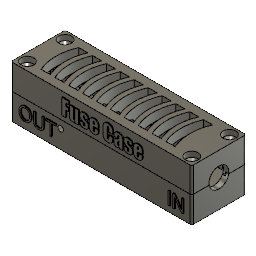
ANL_Fuse_Case (Autodesk Fusion 360 design; units mm, degrees)
Autodesk Fusion 360 part; units mm, degrees
note: some values were not read from the file. Set by a fixed rule: which face or edge a step refers to.
sketch "Skizze1" plane through (0, 0, 0) normal (0, 1, 0) x (1, 0, 0)
  line L0 (50, 15) -> (-50, 15)
  line L1 (-50, 15) -> (-50, -15)
  line L2 (-50, -15) -> (50, -15)
  line L3 (50, -15) -> (50, 15)
  line L4 (50, 15) -> (-50, -15) construction
  line L5 (-50, 15) -> (50, -15) construction
  circle A0 centre (-31, 0) radius 3.1
  line L6 (1.75, 0) -> (22.5, 0)
  line L7 (0, -1.75) -> (0, -22.5)
  circle A1 centre (31, 0) radius 3.1
  dimension "d3" = 30
  dimension "d4" = 100
  dimension "d5" = 6.2
  dimension "d9" = 6.2
  dimension "d10" = 62
  measures "d5" diameter of A0
  measures "d9" diameter of A1
extrude "Extrusion1" add sketch "Skizze1" along normal blind 5 makes body 1
sketch "Skizze3" plane through (0, 5, 0) normal (0, 1, 0) x (-1, 0, 0)
  line L0 (-50, 15) -> (-50, -15)
  line L1 (-50, -15) -> (50, -15)
  line L2 (50, -15) -> (50, 15)
  line L3 (50, 15) -> (-50, 15)
  line L4 (47, -12) -> (-47, -12)
  line L5 (-47, -12) -> (-47, 12)
  line L6 (-47, 12) -> (47, 12)
  line L7 (47, 12) -> (47, -12)
  line L8 (47, -12) -> (-47, 12) construction
  line L9 (-47, -12) -> (47, 12) construction
  circle A0 centre (31, 0) radius 3.1
  circle A1 centre (-31, 0) radius 3.1
  dimension "d17" = 94
  dimension "d18" = 24
extrude "Extrusion3" add sketch "Skizze3" along normal blind 5 contours L0 L1 L2 L3 bodies 1
sketch "Skizze5" plane through (0, 5, 0) normal (0, 1, 0) x (-1, 0, 0)
  line L0 (-47, -12) -> (47, -12)
  line L1 (47, -12) -> (47, 12)
  line L2 (47, 12) -> (-47, 12)
  line L3 (-47, 12) -> (-47, -12)
  circle A0 centre (31, 0) radius 3.1
  circle A1 centre (-31, 0) radius 3.1
  circle A2 centre (31, 0) radius 9
  circle A3 centre (-31, 0) radius 9
  dimension "d25" = 18
  dimension "d26" = 18
  measures "d25" diameter of A2
  measures "d26" diameter of A3
extrude "Extrusion5" add sketch "Skizze5" along normal blind 2 contours A2 | A3 bodies 1
sketch "Skizze6" plane through (0, 0, 0) normal (0, -1, 0) x (1, 0, 0)
  circle A0 centre (-31, 0) radius 3.1
  circle A1 centre (31, 0) radius 3.1
  line L0 (50, -15) -> (50, 15)
  line L1 (50, 15) -> (-50, 15)
  line L2 (-50, 15) -> (-50, -15)
  line L3 (-50, -15) -> (50, -15)
  line L4 (-50, -15) -> (-50, 15)
  line L5 (-50, 15) -> (50, 15)
  line L6 (50, -15) -> (-50, -15)
  line L7 (50, 15) -> (50, -15)
  circle A2 centre (31, 0) radius 3.1
  circle A3 centre (-31, 0) radius 3.1
extrude "Extrusion6" add sketch "Skizze6" along normal blind 3 bodies 1
sketch "Skizze7" plane through (0, -3, 0) normal (0, -1, 0) x (1, 0, 0)
  circle A0 centre (-31, 0) radius 3.1
  circle A1 centre (31, 0) radius 3.1
  line L0 (50, 15) -> (-50, 15)
  line L1 (-50, 15) -> (-50, -15)
  line L2 (-50, -15) -> (50, -15)
  line L3 (50, -15) -> (50, 15)
  line L4 (-33.3094, 4) -> (-35.6188, 0)
  line L5 (-35.6188, 0) -> (-33.3094, -4)
  line L6 (-33.3094, -4) -> (-28.6906, -4)
  line L7 (-28.6906, -4) -> (-26.3812, 0)
  line L8 (-26.3812, 0) -> (-28.6906, 4)
  line L9 (-28.6906, 4) -> (-33.3094, 4)
  line L10 (28.6906, 4) -> (26.3812, 0)
  line L11 (26.3812, 0) -> (28.6906, -4)
  line L12 (28.6906, -4) -> (33.3094, -4)
  line L13 (33.3094, -4) -> (35.6188, 0)
  line L14 (35.6188, 0) -> (33.3094, 4)
  line L15 (33.3094, 4) -> (28.6906, 4)
  dimension "d82" = 8
  dimension "d83" = 8
  measures "d82" distance of L6 L9
  measures "d83" distance of L12 L15
extrude "Extrusion7" cut sketch "Skizze7" against normal blind 5 contours L4 L5 L6 L7 L8 L9 | L10 L11 L12 L13 L14 L15 bodies 1
sketch "Skizze9" plane through (0, 5, 0) normal (0, 1, 0) x (-1, 0, 0)
  circle A0 centre (-31, 0) radius 9
  circle A1 centre (31, 0) radius 9
  line L0 (-47, -12) -> (47, -12)
  line L1 (47, -12) -> (47, 12)
  line L2 (47, 12) -> (-47, 12)
  line L3 (-47, 12) -> (-47, -12)
  line L4 (22, -12) -> (-22, -12)
  line L5 (-22, -12) -> (-22, 12)
  line L6 (-22, 12) -> (22, 12)
  line L7 (22, 12) -> (22, -12)
  line L8 (22, -12) -> (-22, 12) construction
  line L9 (-22, -12) -> (22, 12) construction
  dimension "d35" = 44
extrude "Extrusion9" cut sketch "Skizze9" against normal blind 2 contours L0 L2 L4 L5 L6 L7 bodies 1
sketch "Skizze10" plane through (0, 10, 0) normal (0, 1, 0) x (-1, 0, 0)
  line L0 (-47, 12) -> (47, 12)
  line L1 (47, 12) -> (47, -12)
  line L2 (47, -12) -> (-47, -12)
  line L3 (-47, -12) -> (-47, 12)
  line L4 (50, 15) -> (-50, 15)
  line L5 (-50, 15) -> (-50, -15)
  line L6 (-50, -15) -> (50, -15)
  line L7 (50, -15) -> (50, 15)
  line L8 (48.6, -13.6) -> (-48.6, -13.6)
  line L9 (-48.6, -13.6) -> (-48.6, 13.6)
  line L10 (-48.6, 13.6) -> (48.6, 13.6)
  line L11 (48.6, 13.6) -> (48.6, -13.6)
  line L12 (48.6, -13.6) -> (-48.6, 13.6) construction
  line L13 (-48.6, -13.6) -> (48.6, 13.6) construction
  dimension "d92" = 27.2
  dimension "d93" = 97.2
  measures "d92" distance of L8 L10
  measures "d93" distance of L9 L11
extrude "Extrusion10" add sketch "Skizze10" along normal blind 1.5 contours L4 L5 L6 L7 bodies 1
sketch "Skizze11" plane through (0, 11.5, 0) normal (0, 1, 0) x (-1, 0, 0)
  line L0 (-48.6, 13.6) -> (48.6, 13.6)
  line L1 (48.6, 13.6) -> (48.6, -13.6)
  line L2 (48.6, -13.6) -> (-48.6, -13.6)
  line L3 (-48.6, -13.6) -> (-48.6, 13.6)
  line L4 (50, -15) -> (50, 15)
  line L5 (50, 15) -> (-50, 15)
  line L6 (-50, 15) -> (-50, -15)
  line L7 (-50, -15) -> (50, -15)
  line L8 (50, -15) -> (-50, -15)
  line L9 (-50, -15) -> (-50, 15)
  line L10 (-50, 15) -> (50, 15)
  line L11 (50, 15) -> (50, -15)
  line L12 (50, -15) -> (-50, 15) construction
  line L13 (-50, -15) -> (50, 15) construction
  line L14 (47, -12) -> (-47, -12)
  line L15 (-47, -12) -> (-47, 12)
  line L16 (-47, 12) -> (47, 12)
  line L17 (47, 12) -> (47, -12)
  line L18 (47, -12) -> (-47, 12) construction
  line L19 (-47, -12) -> (47, 12) construction
extrude "Extrusion11" add sketch "Skizze11" along normal blind 9 separate body contours L0 L1 L2 L3 | L4 L5 L6 L7 L8 L9 L10 L11 makes body 2
sketch "Skizze12" plane through (0, 11.5, 0) normal (0, -1, 0) x (1, 0, 0)
  line L0 (-47, 12) -> (47, 12)
  line L1 (47, 12) -> (47, -12)
  line L2 (47, -12) -> (-47, -12)
  line L3 (-47, -12) -> (-47, 12)
  line L4 (50, 15) -> (-50, 15)
  line L5 (-50, 15) -> (-50, -15)
  line L6 (-50, -15) -> (50, -15)
  line L7 (50, -15) -> (50, 15)
  line L8 (-48.25, 13.25) -> (48.25, 13.25)
  line L9 (48.25, 13.25) -> (48.25, -13.25)
  line L10 (48.25, -13.25) -> (-48.25, -13.25)
  line L11 (-48.25, -13.25) -> (-48.25, 13.25)
  line L12 (-48.25, 13.25) -> (48.25, -13.25) construction
  line L13 (48.25, 13.25) -> (-48.25, -13.25) construction
  dimension "d42" = 96.5
  dimension "d94" = 26.5
extrude "Extrusion12" add sketch "Skizze12" along normal blind 1 contours L8 L9 L10 L11 bodies 2
sketch "Skizze13" plane through (-50, 0, 0) normal (-1, 0, 0) x (0, 0, 1)
  line L0 (15, -3) -> (15, 11.5)
  line L1 (15, 11.5) -> (-15, 11.5)
  line L2 (-15, 11.5) -> (-15, -3)
  line L3 (-15, -3) -> (15, -3)
  line L4 (-12, 5) -> (12, 5)
  line L5 (0, 1.75) -> (0, 22.5)
  circle A0 centre (0, 12.5) radius 5.5
  dimension "d45" = 11
  dimension "d46" = 7.5
  measures "d45" diameter of A0
  measures "d46" distance of L4
extrude "Extrusion13" cut sketch "Skizze13" against normal blind 100 contours L1 L5 A0 | L1 L5 A0 | L1 L5 A0 | L1 L5 A0 bodies 1 2
sketch "Skizze14" plane through (0, 5, 0) normal (0, 1, 0) x (-1, 0, 0)
  line L0 (22, -12) -> (47, -12)
  line L1 (47, -12) -> (47, 12)
  line L2 (47, 12) -> (22, 12)
  circle A0 centre (31, 0) radius 9
  arc A1 (47, -7) -> (42, -12) centre (47, -12) ccw
  arc A2 (42, 12) -> (47, 7) centre (47, 12) ccw
  arc A3 (-42, -12) -> (-47, -7) centre (-47, -12) ccw
  line L3 (-47, -12) -> (47, -12)
  line L4 (-47, -5.1235) -> (-47, -12)
  arc A4 (-47, 7) -> (-42, 12) centre (-47, 12) ccw
  line L5 (-47, -12) -> (-47, 12)
  line L6 (-22, 12) -> (-47, 12)
  line L7 (22, 0) -> (22, -12)
  line L8 (22, 12) -> (22, 0)
  dimension "d49" = 5
  dimension "d50" = 5
  dimension "d51" = 5
  dimension "d52" = 5
  measures "d49" radius of A1
  measures "d50" radius of A2
  measures "d51" radius of A3
  measures "d52" radius of A4
extrude "Extrusion14" add sketch "Skizze14" along normal blind 5 contours L0 L1 A1 L3 | L1 L2 A2 | A3 L3 L4 L5 | A4 L5 L6 bodies 1
sketch "Skizze15" plane through (0, 10, 0) normal (0, 1, 0) x (-1, 0, 0)
  line L0 (-47, -4.899) -> (-48.6, -4.899)
  line L1 (-48.6, -4.899) -> (-48.6, -13.6)
  line L2 (-48.6, -13.6) -> (48.6, -13.6)
  line L3 (48.6, -13.6) -> (48.6, -4.899)
  line L4 (48.6, -4.899) -> (47, -4.899)
  line L5 (47, -4.899) -> (47, -7)
  arc A0 (47, -7) -> (42, -12) centre (47, -12) ccw
  line L6 (42, -12) -> (-42, -12)
  arc A1 (-42, -12) -> (-47, -7) centre (-47, -12) ccw
  line L7 (-47, -7) -> (-47, -4.899)
  circle A2 centre (45.4, -10.4) radius 1.6
  line L8 (47, -12) -> (-47, -12)
  line L9 (47, 12) -> (47, -12)
  circle A3 centre (45.4, 10.4) radius 1.6
  line L10 (-47, 12) -> (47, 12)
  circle A4 centre (-45.4, -10.4) radius 1.6
  line L11 (-47, -12) -> (-47, 12)
  circle A5 centre (-45.4, 10.4) radius 1.6
  dimension "d55" = 3.2
  dimension "d56" = 3.2
  dimension "d57" = 3.2
  dimension "d58" = 3.2
  measures "d55" diameter of A2
  measures "d56" diameter of A3
  measures "d57" diameter of A4
  measures "d58" diameter of A5
extrude "Extrusion15" cut sketch "Skizze15" against normal blind 13 contours A5 | A4 | A3 | A2 bodies 1
sketch "Skizze16" plane through (0, -3, 0) normal (0, -1, 0) x (1, 0, 0)
  circle A0 centre (-45.4, 10.4) radius 1.6
  circle A1 centre (45.4, -10.4) radius 1.6
  circle A2 centre (-45.4, -10.4) radius 1.6
  circle A3 centre (45.4, 10.4) radius 1.6
  line L0 (26.3812, 0) -> (28.6906, 4)
  line L1 (28.6906, 4) -> (33.3094, 4)
  line L2 (33.3094, 4) -> (35.6188, 0)
  line L3 (35.6188, 0) -> (33.3094, -4)
  line L4 (33.3094, -4) -> (28.6906, -4)
  line L5 (28.6906, -4) -> (26.3812, 0)
  line L6 (-35.6188, 0) -> (-33.3094, 4)
  line L7 (-33.3094, 4) -> (-28.6906, 4)
  line L8 (-28.6906, 4) -> (-26.3812, 0)
  line L9 (-26.3812, 0) -> (-28.6906, -4)
  line L10 (-28.6906, -4) -> (-33.3094, -4)
  line L11 (-33.3094, -4) -> (-35.6188, 0)
  line L12 (50, 15) -> (-50, 15)
  line L13 (-50, 15) -> (-50, -15)
  line L14 (-50, -15) -> (50, -15)
  line L15 (50, -15) -> (50, 15)
  line L16 (-47.0166, 13.2) -> (-48.6332, 10.4)
  line L17 (-48.6332, 10.4) -> (-47.0166, 7.6)
  line L18 (-47.0166, 7.6) -> (-43.7834, 7.6)
  line L19 (-43.7834, 7.6) -> (-42.1668, 10.4)
  line L20 (-42.1668, 10.4) -> (-43.7834, 13.2)
  line L21 (-43.7834, 13.2) -> (-47.0166, 13.2)
  line L22 (-47.0166, -7.6) -> (-48.6332, -10.4)
  line L23 (-48.6332, -10.4) -> (-47.0166, -13.2)
  line L24 (-47.0166, -13.2) -> (-43.7834, -13.2)
  line L25 (-43.7834, -13.2) -> (-42.1668, -10.4)
  line L26 (-42.1668, -10.4) -> (-43.7834, -7.6)
  line L27 (-43.7834, -7.6) -> (-47.0166, -7.6)
  line L28 (43.7834, -7.6) -> (42.1668, -10.4)
  line L29 (42.1668, -10.4) -> (43.7834, -13.2)
  line L30 (43.7834, -13.2) -> (47.0166, -13.2)
  line L31 (47.0166, -13.2) -> (48.6332, -10.4)
  line L32 (48.6332, -10.4) -> (47.0166, -7.6)
  line L33 (47.0166, -7.6) -> (43.7834, -7.6)
  line L34 (43.7834, 13.2) -> (42.1668, 10.4)
  line L35 (42.1668, 10.4) -> (43.7834, 7.6)
  line L36 (43.7834, 7.6) -> (47.0166, 7.6)
  line L37 (47.0166, 7.6) -> (48.6332, 10.4)
  line L38 (48.6332, 10.4) -> (47.0166, 13.2)
  line L39 (47.0166, 13.2) -> (43.7834, 13.2)
  dimension "d88" = 5.6
  dimension "d89" = 5.6
  dimension "d90" = 5.6
  dimension "d91" = 5.6
  measures "d88" distance of L18 L21
  measures "d89" distance of L24 L27
  measures "d90" distance of L36 L39
  measures "d91" distance of L30 L33
extrude "Extrusion16" cut sketch "Skizze16" against normal blind 3 contours L16 L17 L18 L19 L20 L21 | L22 L23 L24 L25 L26 L27 | L28 L29 L30 L31 L32 L33 | L34 L35 L36 L37 L38 L39 bodies 1
sketch "Skizze17" plane through (0, 20.5, 0) normal (0, 1, 0) x (-1, 0, 0)
  line L0 (-47, 12) -> (47, 12)
  line L1 (47, 12) -> (47, -12)
  line L2 (47, -12) -> (-47, -12)
  line L3 (-47, -12) -> (-47, 12)
  line L4 (50, 15) -> (-50, 15)
  line L5 (-50, 15) -> (-50, -15)
  line L6 (-50, -15) -> (50, -15)
  line L7 (50, -15) -> (50, 15)
extrude "Extrusion17" add sketch "Skizze17" along normal blind 5 contours L0 L1 L2 L3 | L4 L5 L6 L7 bodies 2
sketch "Skizze18" plane through (0, 25.5, 0) normal (0, 1, 0) x (-1, 0, 0)
  line L0 (50, -15) -> (50, 15)
  line L1 (50, 15) -> (-50, 15)
  line L2 (-50, 15) -> (-50, -15)
  line L3 (-50, -15) -> (50, -15)
  circle A0 centre (45.4, 10.4) radius 1.6
  circle A1 centre (45.4, -10.4) radius 1.6
  circle A2 centre (-45.4, 10.4) radius 1.6
  circle A3 centre (-45.4, 10.4) radius 1.6
  circle A4 centre (-45.4, -10.4) radius 1.6
  circle A5 centre (45.4, -10.4) radius 3.5
  circle A6 centre (45.4, 10.4) radius 3.5
  circle A7 centre (-45.4, 10.4) radius 3.5
  circle A8 centre (-45.4, -10.4) radius 3.5
  dimension "d65" = 7
  dimension "d66" = 7
  dimension "d67" = 7
  dimension "d68" = 7
  measures "d65" diameter of A5
  measures "d66" diameter of A6
  measures "d67" diameter of A7
  measures "d68" diameter of A8
extrude "Extrusion18" cut sketch "Skizze18" against normal blind 3 contours A5 | A6 | A7 | A8 bodies 2
extrude "Extrusion19" cut 4 faces at (-45.7325, 25.5, -11.1314) (-45.791, 25.5, 11.0772) (45.009, 25.5, -9.7228) (45.009, 25.5, 11.0772) along direction (0, -1, 0) blind 5 on bodies 2 bodies 2
sketch "Skizze19" plane through (0, 20.5, 0) normal (0, -1, 0) x (1, 0, 0)
  arc A0 (47, -10.4) -> (45.4, -12) centre (45.4, -10.4) ccw
  line L0 (47, -10.4) -> (47, 10.4)
  arc A1 (45.4, 12) -> (47, 10.4) centre (45.4, 10.4) ccw
  line L1 (45.4, 12) -> (-45.4, 12)
  arc A2 (-47, 10.4) -> (-45.4, 12) centre (-45.4, 10.4) ccw
  line L2 (-47, 10.4) -> (-47, -10.4)
  arc A3 (-45.4, -12) -> (-47, -10.4) centre (-45.4, -10.4) ccw
  line L3 (-45.4, -12) -> (45.4, -12)
  arc A4 (-42, -12) -> (-47, -7) centre (-47, -12) ccw
  arc A5 (-47, 7) -> (-42, 12) centre (-47, 12) ccw
  arc A6 (47, -7) -> (42, -12) centre (47, -12) ccw
  arc A7 (42, 12) -> (47, 7) centre (47, 12) ccw
extrude "Extrusion20" add sketch "Skizze19" 4 faces at (46.6857, 20.5, -11.6857) (46.6857, 20.5, 11.6857) (-46.6857, 20.5, -11.6857) (-46.6857, 20.5, 11.6857) along normal blind 10 contours A0 L0 L3 A6 | L0 A1 L1 A7 | L2 A3 L3 A4 | L1 A2 L2 A5 on bodies 2 bodies 2
sketch "Skizze20" plane through (0, 25.5, 0) normal (0, 1, 0) x (-1, 0, 0)
  circle A0 centre (45.4, 10.4) radius 3.5
  circle A1 centre (-45.4, -10.4) radius 3.5
  circle A2 centre (45.4, -10.4) radius 3.5
  circle A3 centre (-45.4, 10.4) radius 3.5
  line L0 (50, -15) -> (50, 15)
  line L1 (50, 15) -> (-50, 15)
  line L2 (-50, 15) -> (-50, -15)
  line L3 (-50, -15) -> (50, -15)
  arc A4 (32.8458, -10.3624) -> (32.8316, 10.3949) centre (9, 0) ccw
  arc A5 (37.8458, -10.3624) -> (37.815, 10.433) centre (14, 0) ccw
  circle A6 centre (31, 0) radius 9
  line L4 (37.8458, -10.3624) -> (32.8458, -10.3624)
  line L5 (37.815, 10.433) -> (32.8316, 10.3949)
  arc A7 (30.1791, -10.3624) -> (30.1483, 10.433) centre (6.3333, 0) ccw
  arc A8 (25.1791, -10.3624) -> (25.165, 10.3949) centre (1.3333, 0) ccw
  line L6 (30.1791, -10.3624) -> (25.1791, -10.3624)
  line L7 (30.1483, 10.433) -> (25.165, 10.3949)
  arc A9 (22.5124, -10.3624) -> (22.4816, 10.433) centre (-1.3333, 0) ccw
  arc A10 (17.5124, -10.3624) -> (17.4983, 10.3949) centre (-6.3333, 0) ccw
  line L8 (22.5124, -10.3624) -> (17.5124, -10.3624)
  line L9 (22.4816, 10.433) -> (17.4983, 10.3949)
  arc A11 (14.8458, -10.3624) -> (14.815, 10.433) centre (-9, 0) ccw
  arc A12 (9.8458, -10.3624) -> (9.8316, 10.3949) centre (-14, 0) ccw
  line L10 (14.8458, -10.3624) -> (9.8458, -10.3624)
  line L11 (14.815, 10.433) -> (9.8316, 10.3949)
  arc A13 (7.1791, -10.3624) -> (7.1483, 10.433) centre (-16.6667, 0) ccw
  arc A14 (2.1791, -10.3624) -> (2.165, 10.3949) centre (-21.6667, 0) ccw
  line L12 (7.1791, -10.3624) -> (2.1791, -10.3624)
  line L13 (7.1483, 10.433) -> (2.165, 10.3949)
  arc A15 (-0.4876, -10.3624) -> (-0.5184, 10.433) centre (-24.3333, 0) ccw
  arc A16 (-5.4876, -10.3624) -> (-5.5017, 10.3949) centre (-29.3333, 0) ccw
  line L14 (-0.4876, -10.3624) -> (-5.4876, -10.3624)
  line L15 (-0.5184, 10.433) -> (-5.5017, 10.3949)
  arc A17 (-8.1542, -10.3624) -> (-8.185, 10.433) centre (-32, 0) ccw
  arc A18 (-13.1542, -10.3624) -> (-13.1684, 10.3949) centre (-37, 0) ccw
  line L16 (-8.1542, -10.3624) -> (-13.1542, -10.3624)
  line L17 (-8.185, 10.433) -> (-13.1684, 10.3949)
  arc A19 (-15.8209, -10.3624) -> (-15.8517, 10.433) centre (-39.6667, 0) ccw
  arc A20 (-20.8209, -10.3624) -> (-20.835, 10.3949) centre (-44.6667, 0) ccw
  line L18 (-15.8209, -10.3624) -> (-20.8209, -10.3624)
  line L19 (-15.8517, 10.433) -> (-20.835, 10.3949)
  arc A21 (-23.4876, -10.3624) -> (-23.5184, 10.433) centre (-47.3333, 0) ccw
  arc A22 (-28.4876, -10.3624) -> (-28.5017, 10.3949) centre (-52.3333, 0) ccw
  line L20 (-23.4876, -10.3624) -> (-28.4876, -10.3624)
  line L21 (-23.5184, 10.433) -> (-28.5017, 10.3949)
  arc A23 (-31.1542, -10.3624) -> (-31.185, 10.433) centre (-55, 0) ccw
  arc A24 (-36.1542, -10.3624) -> (-36.1684, 10.3949) centre (-60, 0) ccw
  line L22 (-31.1542, -10.3624) -> (-36.1542, -10.3624)
  line L23 (-31.185, 10.433) -> (-36.1684, 10.3949)
  dimension "d77" = -69
  dimension "d78" = 0
extrude "Extrusion21" cut sketch "Skizze20" against normal blind 5 contours A4 A5 A6 L4 | A4 A6 | A4 A5 A6 L5 | A6 A7 A8 L6 | A6 A7 A8 | A6 A7 A8 L7 | A6 A9 A10 L8 L9 | A6 A9 | A11 A12 L10 L11 | A13 A14 L12 L13 | A15 A16 L14 L15 | A17 A18 L16 L17 | A19 A20 L18 L19 | A21 A22 L20 L21 | A23 A24 L22 L23 bodies 2
fillet "Abrundung1" radius 1 8 edges at (-50, 4.25, 15) (50, 4.25, 15) (50, 4.25, -15) (-50, 4.25, -15) (-50, 18.5, 15) (50, 18.5, 15) (50, 18.5, -15) (-50, 18.5, -15) on bodies 1 2
sketch "Skizze21" plane through (0, 2, 0) normal (0, -1, 0) x (1, 0, 0)
  circle A0 centre (-31, 0) radius 3.1
  line L0 (-28.6906, 4) -> (-33.3094, 4)
  line L1 (-33.3094, 4) -> (-35.6188, 0)
  line L2 (-35.6188, 0) -> (-33.3094, -4)
  line L3 (-33.3094, -4) -> (-28.6906, -4)
  line L4 (-28.6906, -4) -> (-26.3812, 0)
  line L5 (-26.3812, 0) -> (-28.6906, 4)
  circle A1 centre (-31, 0) radius 2.6
  circle A2 centre (31, 0) radius 2.6
  circle A3 centre (31, 0) radius 3.1
  dimension "d84" = 5.2
  dimension "d85" = 5.2
  measures "d84" diameter of A1
  measures "d85" diameter of A2
extrude "Extrusion22" add sketch "Skizze21" against normal blind 5 contours A0 | A3 bodies 1
sketch "Skizze22" plane through (0, 3, 0) normal (0, 1, 0) x (-1, 0, 0)
  line L0 (22, 12) -> (-22, 12)
  line L1 (-22, 12) -> (-22, -12)
  line L2 (-22, -12) -> (22, -12)
  line L3 (22, -12) -> (22, 12)
  line L4 (22, -12) -> (-22, -12)
  line L5 (-22, -12) -> (-22, -11)
  line L6 (-22, -11) -> (22, -11)
  line L7 (22, -11) -> (22, -12)
  line L8 (22, 12) -> (-22, 12)
  line L9 (-22, 12) -> (-22, 11)
  line L10 (-22, 11) -> (22, 11)
  line L11 (22, 11) -> (22, 12)
  dimension "d95" = 24
  dimension "d96" = 1
  dimension "d97" = 1
  measures "d95" distance of L0 L4
  measures "d96" distance of L4 L6
  measures "d97" distance of L8 L10
extrude "Extrusion23" add sketch "Skizze22" along normal blind 2 contours L0 L1 L3 L8 L9 L10 L11 | L1 L2 L3 L4 L5 L6 L7 bodies 1
sketch "Skizze24" plane through (0, 0, 15) normal (0, 0, 1) x (1, 0, 0)
  line L0 (49, 11.5) -> (49, 25.5)
  line L1 (49, 25.5) -> (-49, 25.5)
  line L2 (-49, 25.5) -> (-49, 11.5)
  line L3 (-49, 11.5) -> (49, 11.5)
  line L4 (-21.3454, 14.0591) -> (23.181, 14.0591) construction
  line L5 (23.181, 14.0591) -> (23.181, 25.0591) construction
  line L6 (23.181, 25.0591) -> (-21.3454, 25.0591) construction
  line L7 (-21.3454, 25.0591) -> (-21.3454, 14.0591) construction
  text T0 "Fuse Case" font "Impact" height 11 align ink ink in box 0 x 0 at (-21.3454, 14.0591) x (1, 0) y (0, 1) spacing 1 height is em
extrude "Extrusion24" add sketch "Skizze24" along normal blind 0.5 text T0 bodies 2
sketch "Skizze25" plane through (0, 7, 0) normal (0, 1, 0) x (-1, 0, 0)
  circle A0 centre (31, 0) radius 2.6
  circle A1 centre (31, 0) radius 9
  line L0 (33.3094, -4) -> (35.6188, 0)
  line L1 (35.6188, 0) -> (33.3094, 4)
  line L2 (33.3094, 4) -> (28.6906, 4)
  line L3 (28.6906, 4) -> (26.3812, 0)
  line L4 (26.3812, 0) -> (28.6906, -4)
  line L5 (28.6906, -4) -> (33.3094, -4)
  line L6 (-28.6906, -4) -> (-26.3812, 0)
  line L7 (-26.3812, 0) -> (-28.6906, 4)
  line L8 (-28.6906, 4) -> (-33.3094, 4)
  line L9 (-33.3094, 4) -> (-35.6188, 0)
  line L10 (-35.6188, 0) -> (-33.3094, -4)
  line L11 (-33.3094, -4) -> (-28.6906, -4)
  dimension "d102" = 8
  dimension "d103" = 8
  measures "d102" distance of L2 L5
  measures "d103" distance of L8 L11
extrude "Extrusion25" cut sketch "Skizze25" against normal blind 5 contours L0 L1 L2 L3 L4 L5 | L6 L7 L8 L9 L10 L11 bodies 1
sketch "Skizze26" plane through (0, -3, 0) normal (0, -1, 0) x (1, 0, 0)
  line L0 (-48.6332, -10.4) -> (-47.0166, -7.6)
  line L1 (-47.0166, -7.6) -> (-43.7834, -7.6)
  line L2 (-43.7834, -7.6) -> (-42.1668, -10.4)
  line L3 (-42.1668, -10.4) -> (-43.7834, -13.2)
  line L4 (-43.7834, -13.2) -> (-47.0166, -13.2)
  line L5 (-47.0166, -13.2) -> (-48.6332, -10.4)
  line L6 (42.1668, 10.4) -> (43.7834, 13.2)
  line L7 (43.7834, 13.2) -> (47.0166, 13.2)
  line L8 (47.0166, 13.2) -> (48.6332, 10.4)
  line L9 (48.6332, 10.4) -> (47.0166, 7.6)
  line L10 (47.0166, 7.6) -> (43.7834, 7.6)
  line L11 (43.7834, 7.6) -> (42.1668, 10.4)
  line L12 (-48.6332, 10.4) -> (-47.0166, 13.2)
  line L13 (-47.0166, 13.2) -> (-43.7834, 13.2)
  line L14 (-43.7834, 13.2) -> (-42.1668, 10.4)
  line L15 (-42.1668, 10.4) -> (-43.7834, 7.6)
  line L16 (-43.7834, 7.6) -> (-47.0166, 7.6)
  line L17 (-47.0166, 7.6) -> (-48.6332, 10.4)
  line L18 (42.1668, -10.4) -> (43.7834, -7.6)
  line L19 (43.7834, -7.6) -> (47.0166, -7.6)
  line L20 (47.0166, -7.6) -> (48.6332, -10.4)
  line L21 (48.6332, -10.4) -> (47.0166, -13.2)
  line L22 (47.0166, -13.2) -> (43.7834, -13.2)
  line L23 (43.7834, -13.2) -> (42.1668, -10.4)
  line L24 (26.3812, 0) -> (28.6906, 4)
  line L25 (28.6906, 4) -> (33.3094, 4)
  line L26 (33.3094, 4) -> (35.6188, 0)
  line L27 (35.6188, 0) -> (33.3094, -4)
  line L28 (33.3094, -4) -> (28.6906, -4)
  line L29 (28.6906, -4) -> (26.3812, 0)
  line L30 (-35.6188, 0) -> (-33.3094, 4)
  line L31 (-33.3094, 4) -> (-28.6906, 4)
  line L32 (-28.6906, 4) -> (-26.3812, 0)
  line L33 (-26.3812, 0) -> (-28.6906, -4)
  line L34 (-28.6906, -4) -> (-33.3094, -4)
  line L35 (-33.3094, -4) -> (-35.6188, 0)
  arc A0 (-50, -14) -> (-49, -15) centre (-49, -14) ccw
  line L36 (-49, -15) -> (49, -15)
  arc A1 (49, -15) -> (50, -14) centre (49, -14) ccw
  line L37 (50, -14) -> (50, 14)
  arc A2 (50, 14) -> (49, 15) centre (49, 14) ccw
  line L38 (49, 15) -> (-49, 15)
  arc A3 (-49, 15) -> (-50, 14) centre (-49, 14) ccw
  line L39 (-50, 14) -> (-50, -14)
  circle A4 centre (-31, 0) radius 2.6
  line L40 (-28.6906, 4) -> (-33.3094, 4)
  line L41 (-33.3094, 4) -> (-35.6188, 0)
  line L42 (-35.6188, 0) -> (-33.3094, -4)
  line L43 (-33.3094, -4) -> (-28.6906, -4)
  line L44 (-28.6906, -4) -> (-26.3812, 0)
  line L45 (-26.3812, 0) -> (-28.6906, 4)
  circle A5 centre (31, 0) radius 2.6
  line L46 (33.3094, 4) -> (28.6906, 4)
  line L47 (28.6906, 4) -> (26.3812, 0)
  line L48 (26.3812, 0) -> (28.6906, -4)
  line L49 (28.6906, -4) -> (33.3094, -4)
  line L50 (33.3094, -4) -> (35.6188, 0)
  line L51 (35.6188, 0) -> (33.3094, 4)
extrude "Extrusion26" add sketch "Skizze26" against normal blind 5 contours L24 L25 L26 L27 L28 L29 L46 L47 L48 L49 L50 L51 | L30 L31 L32 L33 L34 L35 L40 L41 L42 L43 L44 L45 bodies 1
extrude "Extrusion27" cut 2 faces at (26.2119, 7, 3.0233) (-36.0123, 7, 2.635) along direction (0, -1, 0) blind 1 on bodies 1 bodies 1
sketch "Skizze28" plane through (0, 0, 15) normal (0, 0, 1) x (1, 0, 0)
  line L0 (49, -3) -> (49, 11.5)
  line L1 (49, 11.5) -> (-49, 11.5)
  line L2 (-49, 11.5) -> (-49, -3)
  line L3 (-49, -3) -> (49, -3)
  line L4 (37.4033, 0.5851) -> (45.6504, 0.5851) construction
  line L5 (45.6504, 0.5851) -> (45.6504, 10.5851) construction
  line L6 (45.6504, 10.5851) -> (37.4033, 10.5851) construction
  line L7 (37.4033, 10.5851) -> (37.4033, 0.5851) construction
  line L8 (-45.0165, 1.0191) -> (-24.5917, 1.0191) construction
  line L9 (-24.5917, 1.0191) -> (-24.5917, 11.0191) construction
  line L10 (-24.5917, 11.0191) -> (-45.0165, 11.0191) construction
  line L11 (-45.0165, 11.0191) -> (-45.0165, 1.0191) construction
  text T0 "IN" font "Arial" height 10 align ink ink in box 0 x 0 at (37.4033, 0.5851) x (1, 0) y (0, 1) spacing 1 height is em
  text T1 "OUT" font "Arial" height 10 align ink ink in box 0 x 0 at (-45.0165, 1.0191) x (1, 0) y (0, 1) spacing 1 height is em
extrude "Extrusion28" add sketch "Skizze28" along normal blind 0.5 text T0 T1 bodies 1
sketch "Skizze29" plane through (0, 0, -12) normal (0, 0, 1) x (1, 0, 0)
  line L0 (-42, 5) -> (42, 5)
  line L1 (42, 5) -> (42, 10)
  line L2 (42, 10) -> (-42, 10)
  line L3 (-42, 10) -> (-42, 5)
  circle A0 centre (-25, 7.5) radius 1.5
  dimension "d112" = 3
  dimension "d113" = 2.5
  measures "d112" diameter of A0
  measures "d113" distance of L0
extrude "Extrusion29" cut sketch "Skizze29" against normal blind 3 contours A0 bodies 1
sketch "Skizze30" plane through (0, 20.5, 0) normal (0, -1, 0) x (1, 0, 0)
  line L0 (31.185, 10.433) -> (36.1684, 10.3949)
  arc A0 (36.1684, 10.3949) -> (36.1542, -10.3624) centre (60, 0) ccw
  line L1 (36.1542, -10.3624) -> (31.1542, -10.3624)
  arc A1 (31.185, 10.433) -> (31.1542, -10.3624) centre (55, 0) ccw
  line L2 (0.5184, 10.433) -> (5.5017, 10.3949)
  arc A2 (5.5017, 10.3949) -> (5.4876, -10.3624) centre (29.3333, 0) ccw
  line L3 (5.4876, -10.3624) -> (0.4876, -10.3624)
  arc A3 (0.5184, 10.433) -> (0.4876, -10.3624) centre (24.3333, 0) ccw
  line L4 (-22.4816, 10.433) -> (-17.4983, 10.3949)
  arc A4 (-17.4983, 10.3949) -> (-17.5124, -10.3624) centre (6.3333, 0) ccw
  line L5 (-17.5124, -10.3624) -> (-22.5124, -10.3624)
  arc A5 (-22.4816, 10.433) -> (-22.5124, -10.3624) centre (1.3333, 0) ccw
  line L6 (8.185, 10.433) -> (13.1684, 10.3949)
  arc A6 (13.1684, 10.3949) -> (13.1542, -10.3624) centre (37, 0) ccw
  line L7 (13.1542, -10.3624) -> (8.1542, -10.3624)
  arc A7 (8.185, 10.433) -> (8.1542, -10.3624) centre (32, 0) ccw
  line L8 (-37.815, 10.433) -> (-32.8316, 10.3949)
  arc A8 (-32.8316, 10.3949) -> (-32.8458, -10.3624) centre (-9, 0) ccw
  line L9 (-32.8458, -10.3624) -> (-37.8458, -10.3624)
  arc A9 (-37.815, 10.433) -> (-37.8458, -10.3624) centre (-14, 0) ccw
  line L10 (23.5184, 10.433) -> (28.5017, 10.3949)
  arc A10 (28.5017, 10.3949) -> (28.4876, -10.3624) centre (52.3333, 0) ccw
  line L11 (28.4876, -10.3624) -> (23.4876, -10.3624)
  arc A11 (23.5184, 10.433) -> (23.4876, -10.3624) centre (47.3333, 0) ccw
  line L12 (-7.1483, 10.433) -> (-2.165, 10.3949)
  arc A12 (-2.165, 10.3949) -> (-2.1791, -10.3624) centre (21.6667, 0) ccw
  line L13 (-2.1791, -10.3624) -> (-7.1791, -10.3624)
  arc A13 (-7.1483, 10.433) -> (-7.1791, -10.3624) centre (16.6667, 0) ccw
  line L14 (-14.815, 10.433) -> (-9.8316, 10.3949)
  arc A14 (-9.8316, 10.3949) -> (-9.8458, -10.3624) centre (14, 0) ccw
  line L15 (-9.8458, -10.3624) -> (-14.8458, -10.3624)
  arc A15 (-14.815, 10.433) -> (-14.8458, -10.3624) centre (9, 0) ccw
  line L16 (15.8517, 10.433) -> (20.835, 10.3949)
  arc A16 (20.835, 10.3949) -> (20.8209, -10.3624) centre (44.6667, 0) ccw
  line L17 (20.8209, -10.3624) -> (15.8209, -10.3624)
  arc A17 (15.8517, 10.433) -> (15.8209, -10.3624) centre (39.6667, 0) ccw
  line L18 (-30.1483, 10.433) -> (-25.165, 10.3949)
  arc A18 (-25.165, 10.3949) -> (-25.1791, -10.3624) centre (-1.3333, 0) ccw
  line L19 (-25.1791, -10.3624) -> (-30.1791, -10.3624)
  arc A19 (-30.1483, 10.433) -> (-30.1791, -10.3624) centre (-6.3333, 0) ccw
  arc A20 (-47, 7) -> (-42, 12) centre (-47, 12) ccw
  line L20 (-47, 7) -> (-47, -7)
  arc A21 (-42, -12) -> (-47, -7) centre (-47, -12) ccw
  line L21 (-42, -12) -> (42, -12)
  arc A22 (47, -7) -> (42, -12) centre (47, -12) ccw
  line L22 (47, -7) -> (47, 7)
  arc A23 (42, 12) -> (47, 7) centre (47, 12) ccw
  line L23 (42, 12) -> (-42, 12)
  arc A24 (-9.8316, 10.3949) -> (-9.8458, -10.3624) centre (14, 0) ccw
  arc A25 (-50, -14) -> (-49, -15) centre (-49, -14) ccw
  line L24 (-50, -14) -> (-50, 14)
  arc A26 (-49, 15) -> (-50, 14) centre (-49, 14) ccw
  line L25 (-49, 15) -> (49, 15)
  arc A27 (50, 14) -> (49, 15) centre (49, 14) ccw
  line L26 (50, 14) -> (50, -14)
  arc A28 (49, -15) -> (50, -14) centre (49, -14) ccw
  line L27 (49, -15) -> (-49, -15)
  line L28 (36.1684, 10.3949) -> (31.185, 10.433)
  arc A29 (31.185, 10.433) -> (31.1542, -10.3624) centre (55, 0) ccw
  line L29 (31.1542, -10.3624) -> (36.1542, -10.3624)
  arc A30 (36.1684, 10.3949) -> (36.1542, -10.3624) centre (60, 0) ccw
  line L30 (5.5017, 10.3949) -> (0.5184, 10.433)
  arc A31 (0.5184, 10.433) -> (0.4876, -10.3624) centre (24.3333, 0) ccw
  line L31 (0.4876, -10.3624) -> (5.4876, -10.3624)
  arc A32 (5.5017, 10.3949) -> (5.4876, -10.3624) centre (29.3333, 0) ccw
  line L32 (-17.4983, 10.3949) -> (-22.4816, 10.433)
  arc A33 (-22.4816, 10.433) -> (-22.5124, -10.3624) centre (1.3333, 0) ccw
  line L33 (-22.5124, -10.3624) -> (-17.5124, -10.3624)
  arc A34 (-17.4983, 10.3949) -> (-17.5124, -10.3624) centre (6.3333, 0) ccw
  line L34 (13.1684, 10.3949) -> (8.185, 10.433)
  arc A35 (8.185, 10.433) -> (8.1542, -10.3624) centre (32, 0) ccw
  line L35 (8.1542, -10.3624) -> (13.1542, -10.3624)
  arc A36 (13.1684, 10.3949) -> (13.1542, -10.3624) centre (37, 0) ccw
  line L36 (-32.8316, 10.3949) -> (-37.815, 10.433)
  arc A37 (-37.815, 10.433) -> (-37.8458, -10.3624) centre (-14, 0) ccw
  line L37 (-37.8458, -10.3624) -> (-32.8458, -10.3624)
  arc A38 (-32.8316, 10.3949) -> (-32.8458, -10.3624) centre (-9, 0) ccw
  line L38 (28.5017, 10.3949) -> (23.5184, 10.433)
  arc A39 (23.5184, 10.433) -> (23.4876, -10.3624) centre (47.3333, 0) ccw
  line L39 (23.4876, -10.3624) -> (28.4876, -10.3624)
  arc A40 (28.5017, 10.3949) -> (28.4876, -10.3624) centre (52.3333, 0) ccw
  line L40 (-2.165, 10.3949) -> (-7.1483, 10.433)
  arc A41 (-7.1483, 10.433) -> (-7.1791, -10.3624) centre (16.6667, 0) ccw
  line L41 (-7.1791, -10.3624) -> (-2.1791, -10.3624)
  arc A42 (-2.165, 10.3949) -> (-2.1791, -10.3624) centre (21.6667, 0) ccw
  line L42 (-9.8316, 10.3949) -> (-14.815, 10.433)
  arc A43 (-14.815, 10.433) -> (-14.8458, -10.3624) centre (9, 0) ccw
  line L43 (-14.8458, -10.3624) -> (-9.8458, -10.3624)
  arc A44 (-9.8316, 10.3949) -> (-9.8458, -10.3624) centre (14, 0) ccw
  line L44 (20.835, 10.3949) -> (15.8517, 10.433)
  arc A45 (15.8517, 10.433) -> (15.8209, -10.3624) centre (39.6667, 0) ccw
  line L45 (15.8209, -10.3624) -> (20.8209, -10.3624)
  arc A46 (20.835, 10.3949) -> (20.8209, -10.3624) centre (44.6667, 0) ccw
  line L46 (-25.165, 10.3949) -> (-30.1483, 10.433)
  arc A47 (-30.1483, 10.433) -> (-30.1791, -10.3624) centre (-6.3333, 0) ccw
  line L47 (-30.1791, -10.3624) -> (-25.1791, -10.3624)
  arc A48 (-25.165, 10.3949) -> (-25.1791, -10.3624) centre (-1.3333, 0) ccw
  circle A49 centre (-45.4, 10.4) radius 3.5
  circle A50 centre (45.4, -10.4) radius 3.5
  circle A51 centre (-45.4, -10.4) radius 3.5
  circle A52 centre (45.4, 10.4) radius 3.5
  line L48 (-9.8316, 10.3949) -> (-9.8316, 12.0088)
  line L49 (-9.8458, -10.3624) -> (-9.8458, -12)
  line L50 (8.1542, -10.3624) -> (8.1542, -12.0072)
  line L51 (8.185, 10.433) -> (8.185, 12)
extrude "Extrusion30" add sketch "Skizze30" along normal blind 7.5 contours A7 A14 L21 L23 A24 A35 A44 L48 L49 L50 L51 bodies 2
ref_plane "Arbeitsebene1" through (10, 0, 0) normal (1, 0, 0) x (0, 1, 0)
sketch "Skizze32" plane through (10, 0, 0) normal (1, 0, 0) x (0, 0, -1)
  circle A0 centre (6, 18) radius 3
  line L0 (-10.3949, 13) -> (10.3624, 13)
  line L1 (12, 13) -> (12, 20.5)
  line L2 (0, 1.75) -> (0, 22.5)
  circle A1 centre (-6, 18) radius 3
  dimension "d119" = 6
  dimension "d120" = 5
  dimension "d121" = 6
  measures "d119" diameter of A0
  measures "d120" distance of L0
  measures "d121" distance of L1
extrude "Extrusion31" cut sketch "Skizze32" against normal blind 23 bodies 2
sketch "Skizze33" plane through (0, 0, 15) normal (0, 0, 1) x (1, 0, 0)
  line L0 (-32.2429, 8.3194) -> (-31.2956, 8.3194)
  line L1 (-31.2956, 8.3194) -> (-31.2956, 4.1836)
  spline S0 degree 3 poles (-31.2956, 4.1836) (-31.3001, 3.8586) (-31.3082, 3.276) (-31.4688, 2.7169) (-31.5398, 2.4698) knots 0 0 0 0 0.096994 0.173794 0.173794 0.173794 0.173794
  spline S1 degree 3 poles (-31.5398, 2.4698) (-31.6402, 2.2664) (-31.8468, 1.8484) (-32.2263, 1.5766) (-32.4211, 1.4371) knots 0 0 0 0 0.066971 0.137643 0.137643 0.137643 0.137643
  spline S2 degree 3 poles (-32.4211, 1.4371) (-32.6626, 1.3212) (-33.1899, 1.0682) (-33.7758, 1.0493) (-34.0935, 1.0391) knots 0 0 0 0 0.079486 0.17358 0.17358 0.17358 0.17358
  spline S3 degree 3 poles (-34.0935, 1.0391) (-34.4027, 1.048) (-34.9731, 1.0645) (-35.4984, 1.2849) (-35.739, 1.3858) knots 0 0 0 0 0.091841 0.169446 0.169446 0.169446 0.169446
  spline S4 degree 3 poles (-35.739, 1.3858) (-35.9366, 1.5136) (-36.3296, 1.7676) (-36.545, 2.1829) (-36.6521, 2.3892) knots 0 0 0 0 0.069307 0.13777 0.13777 0.13777 0.13777
  spline S5 degree 3 poles (-36.6521, 2.3892) (-36.7315, 2.6464) (-36.9118, 3.2299) (-36.9206, 3.8416) (-36.9255, 4.1836) knots 0 0 0 0 0.080359 0.182334 0.182334 0.182334 0.182334
  line L2 (-36.9255, 4.1836) -> (-36.9255, 8.3194)
  line L3 (-36.9255, 8.3194) -> (-35.9782, 8.3194)
  line L4 (-35.9782, 8.3194) -> (-35.9782, 4.1885)
  spline S6 degree 3 poles (-35.9782, 4.1885) (-35.9773, 3.9167) (-35.9756, 3.4506) (-35.8551, 3.0012) (-35.8049, 2.814) knots 0 0 0 0 0.081109 0.139044 0.139044 0.139044 0.139044
  spline S7 degree 3 poles (-35.8049, 2.814) (-35.7363, 2.6749) (-35.5983, 2.395) (-35.3394, 2.2206) (-35.2092, 2.1329) knots 0 0 0 0 0.04567 0.0919 0.0919 0.0919 0.0919
  spline S8 degree 3 poles (-35.2092, 2.1329) (-35.0551, 2.0632) (-34.7273, 1.9148) (-34.3673, 1.901) (-34.1765, 1.8936) knots 0 0 0 0 0.050249 0.106901 0.106901 0.106901 0.106901
  spline S9 degree 3 poles (-34.1765, 1.8936) (-33.8669, 1.9006) (-33.3198, 1.9129) (-32.8787, 2.2297) (-32.6872, 2.3672) knots 0 0 0 0 0.090258 0.15951 0.15951 0.15951 0.15951
  spline S10 degree 3 poles (-32.6872, 2.3672) (-32.5588, 2.5931) (-32.2406, 3.1525) (-32.242, 3.8015) (-32.2429, 4.1885) knots 0 0 0 0 0.076819 0.190279 0.190279 0.190279 0.190279
  line L5 (-32.2429, 4.1885) -> (-32.2429, 8.3194)
  line L6 (-27.8972, 1.1612) -> (-27.8972, 7.4747)
  line L7 (-27.8972, 7.4747) -> (-30.2556, 7.4747)
  line L8 (-30.2556, 7.4747) -> (-30.2556, 8.3194)
  line L9 (-30.2556, 8.3194) -> (-24.5817, 8.3194)
  line L10 (-24.5817, 8.3194) -> (-24.5817, 7.4747)
  line L11 (-24.5817, 7.4747) -> (-26.9499, 7.4747)
  line L12 (-26.9499, 7.4747) -> (-26.9499, 1.1612)
  line L13 (-26.9499, 1.1612) -> (-27.8972, 1.1612)
  line L14 (40.0208, 0.6051) -> (40.0208, 7.7633)
  line L15 (40.0208, 7.7633) -> (40.9924, 7.7633)
  line L16 (40.9924, 7.7633) -> (44.7522, 2.1432)
  line L17 (44.7522, 2.1432) -> (44.7522, 7.7633)
  line L18 (44.7522, 7.7633) -> (45.6604, 7.7633)
  line L19 (45.6604, 7.7633) -> (45.6604, 0.6051)
  line L20 (45.6604, 0.6051) -> (44.6887, 0.6051)
  line L21 (44.6887, 0.6051) -> (40.929, 6.2301)
  line L22 (40.929, 6.2301) -> (40.929, 0.6051)
  line L23 (40.929, 0.6051) -> (40.0208, 0.6051)
  line L24 (37.4133, 0.6051) -> (37.4133, 7.7633)
  line L25 (37.4133, 7.7633) -> (38.3606, 7.7633)
  line L26 (38.3606, 7.7633) -> (38.3606, 0.6051)
  line L27 (38.3606, 0.6051) -> (37.4133, 0.6051)
  line L28 (49, -3) -> (49, 11.5)
  line L29 (49, 11.5) -> (-49, 11.5)
  line L30 (-49, 11.5) -> (-49, -3)
  line L31 (-49, -3) -> (49, -3)
  spline S11 degree 3 poles (-45.0065, 4.6475) (-44.9789, 5.1957) (-44.9271, 6.2216) (-44.3283, 7.0516) (-44.0495, 7.438) knots 0 0 0 0 0.160666 0.300647 0.300647 0.300647 0.300647
  spline S12 degree 3 poles (-44.0495, 7.438) (-43.7015, 7.7321) (-42.9883, 8.3347) (-42.0561, 8.4085) (-41.5788, 8.4463) knots 0 0 0 0 0.133173 0.272917 0.272917 0.272917 0.272917
  spline S13 degree 3 poles (-41.5788, 8.4463) (-41.259, 8.4281) (-40.6307, 8.3921) (-40.068, 8.1108) (-39.7917, 7.9727) knots 0 0 0 0 0.094979 0.186617 0.186617 0.186617 0.186617
  spline S14 degree 3 poles (-39.7917, 7.9727) (-39.5418, 7.7985) (-39.0394, 7.4484) (-38.7326, 6.9183) (-38.5783, 6.6519) knots 0 0 0 0 0.090184 0.181312 0.181312 0.181312 0.181312
  spline S15 degree 3 poles (-38.5783, 6.6519) (-38.4566, 6.3544) (-38.2047, 5.7389) (-38.1758, 5.0741) (-38.1608, 4.7305) knots 0 0 0 0 0.095662 0.197942 0.197942 0.197942 0.197942
  spline S16 degree 3 poles (-38.1608, 4.7305) (-38.1767, 4.3819) (-38.2076, 3.706) (-38.4722, 3.0837) (-38.6003, 2.7823) knots 0 0 0 0 0.103733 0.201152 0.201152 0.201152 0.201152
  spline S17 degree 3 poles (-38.6003, 2.7823) (-38.7602, 2.5142) (-39.076, 1.985) (-39.5912, 1.6475) (-39.8454, 1.481) knots 0 0 0 0 0.092304 0.182213 0.182213 0.182213 0.182213
  spline S18 degree 3 poles (-39.8454, 1.481) (-40.1199, 1.3521) (-40.6709, 1.0934) (-41.2786, 1.0572) (-41.5837, 1.0391) knots 0 0 0 0 0.09006 0.180823 0.180823 0.180823 0.180823
  spline S19 degree 3 poles (-41.5837, 1.0391) (-41.9088, 1.0577) (-42.5455, 1.0941) (-43.1127, 1.385) (-43.3903, 1.5274) knots 0 0 0 0 0.096478 0.188996 0.188996 0.188996 0.188996
  spline S20 degree 3 poles (-43.3903, 1.5274) (-43.6397, 1.7052) (-44.1391, 2.0614) (-44.4438, 2.5938) (-44.5964, 2.8604) knots 0 0 0 0 0.090699 0.181671 0.181671 0.181671 0.181671
  spline S21 degree 3 poles (-44.5964, 2.8604) (-44.716, 3.1462) (-44.9555, 3.7183) (-44.9895, 4.3376) (-45.0065, 4.6475) knots 0 0 0 0 0.092197 0.184565 0.184565 0.184565 0.184565
  circle A0 centre (-22.4275, 7.085) radius 1.5
  dimension "d124" = 3
  measures "d124" diameter of A0
extrude "Extrusion32" cut sketch "Skizze33" against normal blind 3 contours A0 bodies 1
extrude "Extrusion33" cut 1 faces at (7.3333, 3, 3.6667) along direction (0, -1, 0) blind 1 on bodies 1 bodies 1
extrude "Extrusion35" cut 1 faces at (7.3333, 4, 11) along direction (0, 0, 1) blind 1 on bodies 1 bodies 1
extrude "Extrusion36" cut 1 faces at (7.3333, 4, -11) along direction (0, 0, -1) blind 1 on bodies 1 bodies 1
chamfer "Fase1" distance 1.9 angle 45 4 edges at (-43.9083, 22.5, -10.9786) (-43.9083, 22.5, 9.8214) (46.8917, 22.5, 9.8214) (46.8917, 22.5, -10.9786) on bodies 2
chamfer "Fase2" distance 1.2 angle 45 4 edges at (-43.9083, 0, -9.8214) (-43.9083, 0, 10.9786) (46.8917, 0, -9.8214) (46.8917, 0, 10.9786) on bodies 1
equation "d26 = d25"
equation "d66 = d65"
equation "d67 = d65"
equation "d68 = d65"
equation "d83 = d82"
equation "d89 = d88"
equation "d90 = d88"
equation "d91 = d88"
equation "d97 = d96"
equation "d103 = d102"
named bodies: "bottom", "top"
